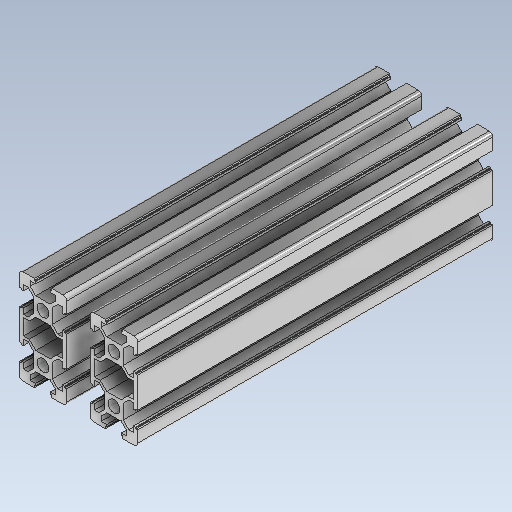
# Autodesk Inventor part: alm ext 2040 150mm
Saved by Autodesk Inventor 2020 (Build 240168000, 168)
## iProperties
Created: 2020-07-11
Part Number: alm ext 2040 150mm
Material: Aluminum 6061
Document SubType Name: Modeling
Designer: Vikki
Density: 2.7 g/cm^3
Appearance: Chrome - Polished
Mass: 228.311 g
Surface Area: 944.953 cm^2
Volume: 84.5595 cm^3
Author: Vikki
Autodesk Inventor part; units mm, degrees
ref_plane "YZ Plane" through (0, 0, 0) normal (1, 0, 0) x (0, 1, 0)
ref_plane "XZ Plane" through (0, 0, 0) normal (0, 1, 0) x (-1, 0, 0)
ref_plane "XY Plane" through (0, 0, 0) normal (0, 0, 1) x (1, 0, 0)
sketch "Sketch1" plane through (0, 0, 0) normal (0, 0, 1) x (1, 0, 0)
  arc A0 (10, 18.5) -> (8.5, 20) centre (8.5, 18.5) ccw projected
  line L0 (3.6, 20) -> (8.5, 20) projected
  line L1 (3.6, 19.3) -> (3.6, 20) projected
  arc A1 (3.4, 19.1) -> (3.6, 19.3) centre (3.4, 19.3) ccw projected
  line L2 (3.1, 19.1) -> (3.4, 19.1) projected
  line L3 (3.1, 18.2) -> (3.1, 19.1) projected
  line L4 (5.45, 18.2) -> (3.1, 18.2) projected
  line L5 (5.45, 16.2985) -> (5.45, 18.2) projected
  line L6 (3.0515, 13.9) -> (5.45, 16.2985) projected
  line L7 (-3.0515, 13.9) -> (3.0515, 13.9) projected
  line L8 (-5.45, 16.2985) -> (-3.0515, 13.9) projected
  line L9 (-5.45, 18.2) -> (-5.45, 16.2985) projected
  line L10 (-3.1, 18.2) -> (-5.45, 18.2) projected
  line L11 (-3.1, 19.1) -> (-3.1, 18.2) projected
  line L12 (-3.4, 19.1) -> (-3.1, 19.1) projected
  arc A2 (-3.6, 19.3) -> (-3.4, 19.1) centre (-3.4, 19.3) ccw projected
  line L13 (-3.6, 20) -> (-3.6, 19.3) projected
  line L14 (-8.5, 20) -> (-3.6, 20) projected
  arc A3 (-8.5, 20) -> (-10, 18.5) centre (-8.5, 18.5) ccw projected
  line L15 (-10, 13.6) -> (-10, 18.5) projected
  line L16 (-9.3, 13.6) -> (-10, 13.6) projected
  arc A4 (-9.1, 13.4) -> (-9.3, 13.6) centre (-9.3, 13.4) ccw projected
  line L17 (-9.1, 13.1) -> (-9.1, 13.4) projected
  line L18 (-8.2, 13.1) -> (-9.1, 13.1) projected
  line L19 (-8.2, 15.45) -> (-8.2, 13.1) projected
  line L20 (-6.2985, 15.45) -> (-8.2, 15.45) projected
  line L21 (-3.9485, 13.1) -> (-6.2985, 15.45) projected
  line L22 (-3.9485, 6.9) -> (-3.9485, 13.1) projected
  line L23 (-6.2985, 4.55) -> (-3.9485, 6.9) projected
  line L24 (-8.2, 4.55) -> (-6.2985, 4.55) projected
  line L25 (-8.2, 6.9) -> (-8.2, 4.55) projected
  line L26 (-9.1, 6.9) -> (-8.2, 6.9) projected
  line L27 (-9.1, 6.6) -> (-9.1, 6.9) projected
  arc A5 (-9.3, 6.4) -> (-9.1, 6.6) centre (-9.3, 6.6) ccw projected
  line L28 (-10, 6.4) -> (-9.3, 6.4) projected
  line L29 (-10, -6.4) -> (-10, 6.4) projected
  line L30 (-9.3, -6.4) -> (-10, -6.4) projected
  arc A6 (-9.1, -6.6) -> (-9.3, -6.4) centre (-9.3, -6.6) ccw projected
  line L31 (-9.1, -6.9) -> (-9.1, -6.6) projected
  line L32 (-8.2, -6.9) -> (-9.1, -6.9) projected
  line L33 (-8.2, -4.55) -> (-8.2, -6.9) projected
  line L34 (-6.2985, -4.55) -> (-8.2, -4.55) projected
  line L35 (-3.9485, -6.9) -> (-6.2985, -4.55) projected
  line L36 (-3.9485, -13.1) -> (-3.9485, -6.9) projected
  line L37 (-6.2985, -15.45) -> (-3.9485, -13.1) projected
  line L38 (-8.2, -15.45) -> (-6.2985, -15.45) projected
  line L39 (-8.2, -13.1) -> (-8.2, -15.45) projected
  line L40 (-9.1, -13.1) -> (-8.2, -13.1) projected
  line L41 (-9.1, -13.4) -> (-9.1, -13.1) projected
  arc A7 (-9.3, -13.6) -> (-9.1, -13.4) centre (-9.3, -13.4) ccw projected
  line L42 (-10, -13.6) -> (-9.3, -13.6) projected
  line L43 (-10, -18.5) -> (-10, -13.6) projected
  arc A8 (-10, -18.5) -> (-8.5, -20) centre (-8.5, -18.5) ccw projected
  line L44 (-3.6, -20) -> (-8.5, -20) projected
  line L45 (-3.6, -19.3) -> (-3.6, -20) projected
  arc A9 (-3.4, -19.1) -> (-3.6, -19.3) centre (-3.4, -19.3) ccw projected
  line L46 (-3.1, -19.1) -> (-3.4, -19.1) projected
  line L47 (-3.1, -18.2) -> (-3.1, -19.1) projected
  line L48 (-5.45, -18.2) -> (-3.1, -18.2) projected
  line L49 (-5.45, -16.2985) -> (-5.45, -18.2) projected
  line L50 (-3.0515, -13.9) -> (-5.45, -16.2985) projected
  line L51 (3.0515, -13.9) -> (-3.0515, -13.9) projected
  line L52 (5.45, -16.2985) -> (3.0515, -13.9) projected
  line L53 (5.45, -18.2) -> (5.45, -16.2985) projected
  line L54 (3.1, -18.2) -> (5.45, -18.2) projected
  line L55 (3.1, -19.1) -> (3.1, -18.2) projected
  line L56 (3.4, -19.1) -> (3.1, -19.1) projected
  arc A10 (3.6, -19.3) -> (3.4, -19.1) centre (3.4, -19.3) ccw projected
  line L57 (3.6, -20) -> (3.6, -19.3) projected
  line L58 (8.5, -20) -> (3.6, -20) projected
  arc A11 (8.5, -20) -> (10, -18.5) centre (8.5, -18.5) ccw projected
  line L59 (10, -13.6) -> (10, -18.5) projected
  line L60 (9.3, -13.6) -> (10, -13.6) projected
  arc A12 (9.1, -13.4) -> (9.3, -13.6) centre (9.3, -13.4) ccw projected
  line L61 (9.1, -13.1) -> (9.1, -13.4) projected
  line L62 (8.2, -13.1) -> (9.1, -13.1) projected
  line L63 (8.2, -15.45) -> (8.2, -13.1) projected
  line L64 (6.2985, -15.45) -> (8.2, -15.45) projected
  line L65 (3.9, -13.0515) -> (6.2985, -15.45) projected
  line L66 (3.9, -6.9485) -> (3.9, -13.0515) projected
  line L67 (6.2985, -4.55) -> (3.9, -6.9485) projected
  line L68 (8.2, -4.55) -> (6.2985, -4.55) projected
  line L69 (8.2, -6.9) -> (8.2, -4.55) projected
  line L70 (9.1, -6.9) -> (8.2, -6.9) projected
  line L71 (9.1, -6.6) -> (9.1, -6.9) projected
  arc A13 (9.3, -6.4) -> (9.1, -6.6) centre (9.3, -6.6) ccw projected
  line L72 (10, -6.4) -> (9.3, -6.4) projected
  line L73 (10, 6.4) -> (10, -6.4) projected
  line L74 (9.3, 6.4) -> (10, 6.4) projected
  arc A14 (9.1, 6.6) -> (9.3, 6.4) centre (9.3, 6.6) ccw projected
  line L75 (9.1, 6.9) -> (9.1, 6.6) projected
  line L76 (8.2, 6.9) -> (9.1, 6.9) projected
  line L77 (8.2, 4.55) -> (8.2, 6.9) projected
  line L78 (6.2985, 4.55) -> (8.2, 4.55) projected
  line L79 (3.9, 6.9485) -> (6.2985, 4.55) projected
  line L80 (3.9, 13.0515) -> (3.9, 6.9485) projected
  line L81 (6.2985, 15.45) -> (3.9, 13.0515) projected
  line L82 (8.2, 15.45) -> (6.2985, 15.45) projected
  line L83 (8.2, 13.1) -> (8.2, 15.45) projected
  line L84 (9.1, 13.1) -> (8.2, 13.1) projected
  line L85 (9.1, 13.4) -> (9.1, 13.1) projected
  arc A15 (9.3, 13.6) -> (9.1, 13.4) centre (9.3, 13.4) ccw projected
  line L86 (10, 13.6) -> (9.3, 13.6) projected
  line L87 (10, 18.5) -> (10, 13.6) projected
  line L88 (5.8015, -3.35) -> (8.2, -3.35) projected
  line L89 (3.0515, -6.1) -> (5.8015, -3.35) projected
  line L90 (-3.0515, -6.1) -> (3.0515, -6.1) projected
  line L91 (-5.8015, -3.35) -> (-3.0515, -6.1) projected
  line L92 (-8.2, -3.35) -> (-5.8015, -3.35) projected
  line L93 (-8.2, 3.35) -> (-8.2, -3.35) projected
  line L94 (-5.8015, 3.35) -> (-8.2, 3.35) projected
  line L95 (-3.0515, 6.1) -> (-5.8015, 3.35) projected
  line L96 (3.0515, 6.1) -> (-3.0515, 6.1) projected
  line L97 (5.8015, 3.35) -> (3.0515, 6.1) projected
  line L98 (8.2, 3.35) -> (5.8015, 3.35) projected
  line L99 (8.2, -3.35) -> (8.2, 3.35) projected
  circle A16 centre (0, 10) radius 2.5 projected
  circle A17 centre (0, -10) radius 2.5 projected
  point P0 (0, 0)
extrude "Extrusion1" add sketch "Sketch1" against normal blind 150
pattern_linear "Rectangular Pattern1" count 2 spacing 30 along (-1, 0, 0) of "Extrusion1"
body "Solid1"
